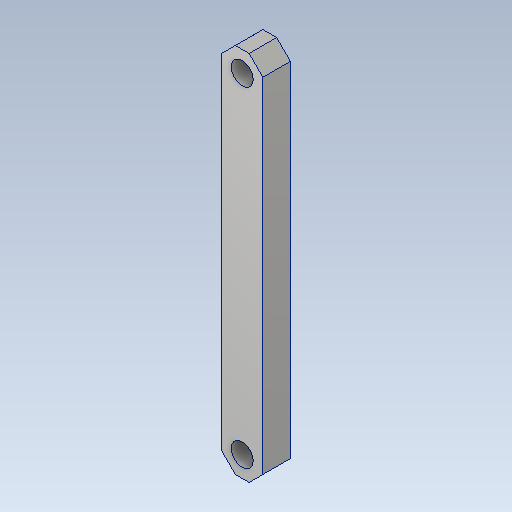
# Autodesk Inventor part: 큰모터서포터
Saved by Autodesk Inventor 2020 (Build 240168000, 168)
## iProperties
Created: 2021-07-06
Part Number: 큰모터서포터
Material: 알루미늄 6061
Document SubType Name: Modeling
Designer: user
Density: 2.7 g/cm^3
Appearance: 알루미늄 - 평지
Mass: 3.23908 g
Surface Area: 11.4151 cm^2
Volume: 1.19966 cm^3
Author: user
Autodesk Inventor part; units mm, degrees
ref_plane "YZ Plane" through (0, 0, 0) normal (1, 0, 0) x (0, 1, 0)
ref_plane "XZ Plane" through (0, 0, 0) normal (0, 1, 0) x (-1, 0, 0)
ref_plane "XY Plane" through (0, 0, 0) normal (0, 0, 1) x (1, 0, 0)
sketch "스케치1" plane through (0, 0, 0) normal (0, 0, 1) x (1, 0, 0)
  line L0 (-3, 27) -> (3, 27)
  line L1 (3, 27) -> (3, -27)
  line L2 (3, -27) -> (-3, -27)
  line L3 (-3, -27) -> (-3, 27)
  point P0 (0, 0)
  dimension "d0" = 6
  dimension "d1" = 54
  dimension "d3" = 3
  dimension "d4" = 27
  constraints: 8 end point, 2 parallel, 1 horizontal, 1 perpendicular
  measures "d0" distance of L1.end L2.end
  measures "d1" distance of L0.end L1.end
  measures "d3" distance from line of L3 point (0, 0)
  measures "d4" distance from line of point (0, 0) L0
extrude "돌출1" add sketch "스케치1" along normal blind 4
sketch "스케치2" plane through (0, 0, 4) normal (0, 0, 1) x (1, 0, 0)
  line L0 (3, 27) -> (-3, 27) projected
  line L1 (-3, 27) -> (-3, -27) projected
  line L2 (-3, -27) -> (3, -27) projected
  line L3 (3, -27) -> (3, 27) projected
  circle A0 centre (0, 24) radius 1.6
  circle A1 centre (0, -24) radius 1.6
  point P0 (0, 0)
  dimension "d7" = 3.2
  dimension "d8" = 3.2
  dimension "d9" = 3
  dimension "d10" = 3
  dimension "d11" = 3
  dimension "d12" = 3
  constraints: 2 centre point
  measures "d7" diameter of A0
  measures "d8" diameter of A1
  measures "d9" distance from line of L2 A1.centre
  measures "d10" distance from line of A1.centre L3
  measures "d11" distance from line of L3 A0.centre
  measures "d12" distance from line of L0 A0.centre
extrude "돌출2" cut sketch "스케치2" against normal up to next contours A0 | A1
chamfer "모따기1" distance 2 angle 45 4 edges at (3, 27, 2) (-3, 27, 2) (-3, -27, 2) (3, -27, 2)
equation "\"d4\" = 0.5 * d1"
